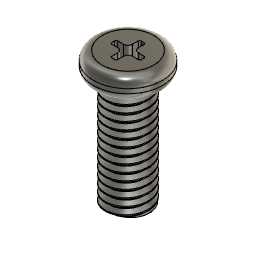
Screw_M3_7.5mm (Autodesk Fusion 360 design; units mm, degrees)
Autodesk Fusion 360 part; units mm, degrees
sketch "スケッチ1" plane through (0, 0, 0) normal (0, 0, 1) x (1, 0, 0)
  circle A0 centre (0, 0) radius 1.5
  dimension "d1" = 3
  constraint coincident A0.centre origin
  measures "d1" diameter of A0
extrude "押し出し1" add sketch "スケッチ1" along normal blind 7.5 makes body 1
thread "ねじ1" "ISO Metric profile 3.0 M3x0.5 6g" major diameter 2.927 minor diameter 2.3555 pitch 0.5 angle 60 modelled right hand crest width 0.0713 on face at (1.4925, -0.1494, 5) crest through (1.4635, 0, -0.125) on bodies 1
sketch "スケッチ2" plane through (0, 0, 7.5) normal (0, 0, 1) x (-1, 0, 0)
  spline S0 degree 3 poles (0.634, -1.319) (0.7937, -1.2229) (0.9334, -1.097) (1.1516, -0.8035) (1.2301, -0.6403) (1.317, -0.2994) (1.3272, -0.1257) (1.2801, 0.209) (1.2259, 0.367) (1.0868, 0.6046) (1.019, 0.6916) (0.864, 0.8428) (0.7781, 0.9068) (0.6847, 0.9583) knots 0 0 0 0 0.055923 0.055923 0.109803 0.109803 0.161639 0.161639 0.211432 0.211432 0.244511 0.244511 0.276632 0.276632 0.276632 0.276632
  arc A0 (0.6847, 0.9583) -> (-0.6847, 0.9583) centre (0, 0) ccw
  spline S1 degree 3 poles (-0.6847, 0.9583) (-0.821, 0.8831) (-0.941, 0.7816) (-1.1406, 0.5335) (-1.2163, 0.3878) (-1.3109, 0.0692) (-1.3263, -0.1013) (-1.2915, -0.4458) (-1.239, -0.6161) (-1.0965, -0.8832) (-1.0222, -0.9858) (-0.8463, -1.1711) (-0.7449, -1.2523) (-0.634, -1.319) knots 0 0 0 0 0.046698 0.046698 0.095434 0.095434 0.146206 0.146206 0.199015 0.199015 0.236706 0.236706 0.275362 0.275362 0.275362 0.275362
  arc A1 (-0.634, -1.319) -> (0.634, -1.319) centre (0, 0) ccw
  circle A2 centre (0, 0) radius 2.35
  dimension "d4" = 4.7
  constraint concentric A0 A2
  measures "d4" diameter of A2
extrude "押し出し2" add sketch "スケッチ2" along normal blind 1.5 separate body contours S0 A0 S1 A1 | A2 makes body 2
fillet "フィレット1" radius 0.6 2 edges at (2.191, 0.8498, 9) (2.191, 0.8498, 7.5) on bodies 2
sketch "スケッチ3" plane through (0, 0, 9) normal (0, 0, 1) x (-1, 0, 0)
  circle A0 centre (0, 0) radius 1.75
  line L0 (-1, 0) -> (-1, -0.1)
  line L1 (-0.9, -0.2) -> (-0.5, -0.2)
  line L2 (-0.2, -0.5) -> (-0.2, -0.9)
  line L3 (-0.1, -1) -> (0.1, -1)
  line L4 (0.2, -0.9) -> (0.2, -0.5)
  line L5 (0.5, -0.2) -> (0.9, -0.2)
  line L6 (1, -0.1) -> (1, 0.1)
  line L7 (0.9, 0.2) -> (0.5, 0.2)
  line L8 (0.2, 0.5) -> (0.2, 0.9)
  line L9 (0.1, 1) -> (-0.1, 1)
  line L10 (-0.2, 0.9) -> (-0.2, 0.5)
  line L11 (-0.5, 0.2) -> (-0.9, 0.2)
  line L12 (-1, 0.1) -> (-1, 0)
  arc A1 (0.5, -0.2) -> (0.2, -0.5) centre (0.5, -0.5) ccw
  arc A2 (-0.2, -0.5) -> (-0.5, -0.2) centre (-0.5, -0.5) ccw
  arc A3 (-0.5, 0.2) -> (-0.2, 0.5) centre (-0.5, 0.5) ccw
  arc A4 (0.2, 0.5) -> (0.5, 0.2) centre (0.5, 0.5) ccw
  arc A5 (0.9, -0.2) -> (1, -0.1) centre (0.9, -0.1) ccw
  arc A6 (1, 0.1) -> (0.9, 0.2) centre (0.9, 0.1) ccw
  arc A7 (0.1, -1) -> (0.2, -0.9) centre (0.1, -0.9) ccw
  arc A8 (-0.2, -0.9) -> (-0.1, -1) centre (-0.1, -0.9) ccw
  arc A9 (-1, -0.1) -> (-0.9, -0.2) centre (-0.9, -0.1) ccw
  arc A10 (-0.9, 0.2) -> (-1, 0.1) centre (-0.9, 0.1) ccw
  arc A11 (-0.1, 1) -> (-0.2, 0.9) centre (-0.1, 0.9) ccw
  arc A12 (0.2, 0.9) -> (0.1, 1) centre (0.1, 0.9) ccw
  dimension "d8" = 0.3
  dimension "d9" = 0.3
  dimension "d10" = 0.3
  dimension "d11" = 0.1
  constraint vertical L0
  constraint perpendicular L0 L1
  constraint perpendicular L1 L2
  constraint perpendicular L2 L3
  constraint perpendicular L3 L4
  constraint perpendicular L2 L5
  constraint perpendicular L3 L6
  constraint perpendicular L2 L7
  constraint perpendicular L3 L8
  constraint perpendicular L2 L9
  constraint perpendicular L9 L10
  constraint perpendicular L10 L11
  constraint perpendicular L11 L12
  constraint tangent L4 A1
  constraint tangent L5 A1
  constraint tangent L1 A2
  constraint tangent L2 A2
  constraint tangent L10 A3
  constraint tangent L11 A3
  constraint equal A2 A3
  constraint tangent L7 A4
  constraint tangent L8 A4
  constraint tangent L5 A5
  constraint tangent L6 A5
  constraint tangent L6 A6
  constraint tangent L7 A6
  constraint equal A5 A6
  constraint tangent L3 A7
  constraint tangent L4 A7
  constraint equal A5 A7
  constraint tangent L2 A8
  constraint tangent L3 A8
  constraint equal A5 A8
  constraint tangent L0 A9
  constraint tangent L1 A9
  constraint equal A5 A9
  constraint tangent L11 A10
  constraint tangent L12 A10
  constraint equal A5 A10
  constraint tangent L9 A11
  constraint tangent L10 A11
  constraint equal A5 A11
  constraint tangent L8 A12
  constraint tangent L9 A12
  constraint equal A5 A12
  measures "d8" radius of A1
  measures "d9" radius of A2
  measures "d10" radius of A4
  measures "d11" radius of A5
extrude "押し出し3" cut sketch "スケッチ3" against normal blind 1 contours L0 L1 L2 L3 L4 L5 L6 L7 L8 L9 L10 L11 L12 A1 A2 A3 A4 A5 A6 A7 A8 A9 A10 A11 A12 bodies 2
